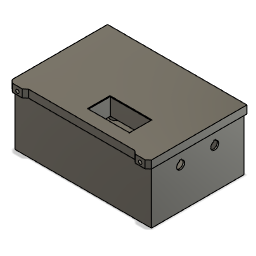
dcdc_ser_v5 (Autodesk Fusion 360 design; units mm, degrees)
Autodesk Fusion 360 part; units mm, degrees
sketch "Skizze1" plane through (0, 0, 0) normal (0, 1, 0) x (1, 0, 0)
  line L0 (0, 0) -> (100, 0) construction
  line L1 (100, 0) -> (100, -64) construction
  line L2 (100, -64) -> (0, -64) construction
  line L3 (0, -64) -> (0, 0) construction
  line L4 (0, 0) -> (100, -64) construction
  circle A0 centre (0, 0) radius 2
  circle A1 centre (0, 0) radius 5
  circle A2 centre (100, 0) radius 5
  circle A3 centre (100, 0) radius 2
  circle A4 centre (0, -64) radius 5
  circle A5 centre (0, -64) radius 2
  circle A6 centre (100, -64) radius 5
  circle A7 centre (100, -64) radius 2
  line L5 (-15, 14) -> (115, 14)
  line L6 (115, 14) -> (115, -78)
  line L7 (115, -78) -> (-15, -78)
  line L8 (-15, -78) -> (-15, 14)
  line L9 (-15, 14) -> (115, -78) construction
  line L10 (115, 14) -> (-15, -78) construction
  line L11 (116.5, -79.5) -> (-16.5, -79.5)
  line L12 (-16.5, -79.5) -> (-16.5, 15.5)
  line L13 (-16.5, 15.5) -> (116.5, 15.5)
  line L14 (116.5, 15.5) -> (116.5, -79.5)
  point P0 (50, -32)
  dimension "d1" = 100
  dimension "d2" = 64
  dimension "d3" = 4
  dimension "d4" = 10
  dimension "d7" = 100
  dimension "d8" = -64
  dimension "d9" = 130
  dimension "d10" = 92
  dimension "d11" = -1.5
  constraint horizontal L0
  constraint vertical L1
  constraint horizontal L2
  constraint vertical L3
  constraint coincident L0.start L3.end
  constraint horizontal L5
  constraint perpendicular L5 L6
  constraint parallel L5 L7
  constraint parallel L6 L8
  constraint coincident L9 P0
  constraint coincident L10 P0
  constraint midpoint L4 P0
  measures "d1" distance of L0.start L0.end
  measures "d2" distance of L0.start L2.end
  measures "d3" diameter of A0
  measures "d4" diameter of A1
  measures "d9" distance of L6.end L7.end
  measures "d10" distance of L5.end L6.end
extrude "Extrusion1" add sketch "Skizze1" against normal blind 1 contours A0 | A1 | A2 | A3 | A4 | A5 | A6 | A7 | L5 L6 L7 L8 | L11 L12 L13 L14 makes body 1
extrude "Extrusion2" add sketch "Skizze1" along normal blind 5 contours A1 | A2 | A4 | A6 bodies 1
extrude "Extrusion3" add sketch "Skizze1" along normal blind 60 contours L11 L12 L13 L14 bodies 1
sketch "Skizze2" plane through (116.5, 0, 0) normal (1, 0, 0) x (0, 0, -1)
  line L0 (-79.5, 60) -> (-79.5, -1)
  line L1 (-79.5, -1) -> (15.5, -1)
  line L2 (15.5, -1) -> (15.5, 60)
  line L3 (15.5, 60) -> (-79.5, 60)
  line L4 (-79.5, 60) -> (15.5, 60) construction
  line L5 (15.5, 60) -> (15.5, 40) construction
  line L6 (15.5, 40) -> (-79.5, 40) construction
  line L7 (-79.5, 40) -> (-79.5, 60) construction
  circle A0 centre (-32, 40) radius 17.5 construction
  line L8 (-49.5, 40) -> (-49.5, 44.1) construction
  line L9 (-14.5, 40) -> (-14.5, 44.1) construction
  line L10 (-48.5, 44.85) -> (-50.5, 44.85)
  line L11 (-50.5, 44.85) -> (-50.5, 43.35)
  line L12 (-49.5, 43.35) -> (-48.5, 43.35)
  line L13 (-48.5, 43.35) -> (-48.5, 44.85)
  line L14 (-48.5, 44.85) -> (-50.5, 43.35) construction
  line L15 (-50.5, 44.85) -> (-48.5, 43.35) construction
  line L16 (-13.5, 44.85) -> (-15.5, 44.85)
  line L17 (-15.5, 44.85) -> (-15.5, 43.35)
  line L18 (-14.8236, 43.35) -> (-13.5, 43.35)
  line L19 (-13.5, 43.35) -> (-13.5, 44.85)
  line L20 (-13.5, 44.85) -> (-15.5, 43.35) construction
  line L21 (-15.5, 44.85) -> (-13.5, 43.35) construction
  arc A1 (-50.5, 43.9762) -> (-49.5, 44.1) centre (-49.5, 40) ccw
  arc A2 (-15.5, 43.9762) -> (-14.9803, 44.0718) centre (-14.5, 40) ccw
  point P0 (-49.5, 44.1)
  point P1 (-14.5, 44.1)
  dimension "d18" = 20
  dimension "d19" = 35
  dimension "d20" = 8.2
  dimension "d21" = 8.2
  dimension "d22" = 2
  dimension "d23" = 1.5
  dimension "d24" = 2
  dimension "d25" = 1.5
  constraint horizontal L4
  constraint vertical L5
  constraint horizontal L6
  constraint vertical L7
  constraint coincident L2 L5.end
  constraint coincident L0.start L3.end
  constraint midpoint L6 A0.centre
  constraint coincident A0 L8.start
  constraint coincident L6 L8.start
  constraint coincident A0 L9.start
  constraint coincident L6 L9.start
  constraint coincident L8.start A1.centre
  constraint tangent A0 L8
  constraint perpendicular L6 L8
  constraint coincident L9.start A2.centre
  constraint coincident P1 A2
  constraint tangent A0 L9
  constraint perpendicular L6 L9
  constraint horizontal L10
  constraint perpendicular L10 L11
  constraint parallel L10 L12
  constraint parallel L11 L13
  constraint coincident L14 P0
  constraint coincident L15 P0
  constraint coincident P0 L8.end
  constraint horizontal L16
  constraint perpendicular L16 L17
  constraint parallel L16 L18
  constraint parallel L17 L19
  constraint coincident L20 P1
  constraint coincident L21 P1
  constraint coincident P1 L9.end
  constraint coincident L8 L12.start
  constraint coincident L11 A1.start
  constraint coincident A0 L18.start
  constraint coincident A0 A2.end
  constraint coincident L17 A2.start
  measures "d18" distance of L0.start L6.end
  measures "d19" diameter of A0
  measures "d20" diameter of A1
  measures "d21" diameter of A2
  measures "d22" distance of L11.end L12.end
  measures "d23" distance of L10.end L11.end
  measures "d24" distance of L17.end L18.end
  measures "d25" distance of L16.end L17.end
extrude "Extrusion4" cut sketch "Skizze2" against normal blind 6 contours L10 L11 L13 A1 | L16 L17 L19 A2 bodies 1
sketch "Skizze3" plane through (-16.5, 0, 0) normal (-1, 0, 0) x (0, 0, 1)
  line L0 (-15.5, 60) -> (-15.5, -1)
  line L1 (-15.5, -1) -> (79.5, -1)
  line L2 (79.5, -1) -> (79.5, 60)
  line L3 (79.5, 60) -> (-15.5, 60)
  line L4 (14.5, 40) -> (14.5, 44.1)
  circle A0 centre (14.5, 43.5) radius 1 construction
  line L5 (13.5103, 43.3571) -> (14.5, 44.5)
  line L6 (15.4897, 43.3571) -> (14.5, 44.5)
  arc A1 (13.5103, 43.3571) -> (14.5, 43.5) centre (14.5, 40) ccw
  arc A2 (13.5103, 23.3571) -> (14.5, 23.5) centre (14.5, 20) ccw
  line L7 (15.4897, 23.3571) -> (14.5, 24.5)
  line L8 (13.5103, 23.3571) -> (14.5, 24.5)
  line L9 (14.4549, 36.5003) -> (14.5, 23.5) construction
  line L10 (14.4774, 30.0001) -> (79.5, 30.0001) construction
  circle A3 centre (46.9887, 30.0001) radius 9
  line L11 (56.9887, 31.0001) -> (54.9887, 31.0001)
  line L12 (54.9887, 31.0001) -> (54.9887, 29.0001)
  line L13 (55.933, 29.0001) -> (56.9887, 29.0001)
  line L14 (56.9887, 29.0001) -> (56.9887, 31.0001)
  line L15 (56.9887, 31.0001) -> (54.9887, 29.0001) construction
  line L16 (54.9887, 31.0001) -> (56.9887, 29.0001) construction
  line L17 (38.0445, 29.0001) -> (36.9887, 29.0001)
  line L18 (36.9887, 29.0001) -> (36.9887, 31.0001)
  line L19 (36.9887, 31.0001) -> (38.9887, 31.0001)
  line L20 (38.9887, 31.0001) -> (38.9887, 29.0001)
  line L21 (38.9887, 29.0001) -> (36.9887, 31.0001) construction
  line L22 (36.9887, 29.0001) -> (38.9887, 31.0001) construction
  line L23 (38.0445, 29.0001) -> (38.9887, 29.9444)
  line L24 (55.933, 29.0001) -> (54.9887, 30.0001)
  point P0 (14.5, 40)
  point P1 (14.5, 44.1)
  point P2 (55.9887, 30.0001)
  point P3 (37.9887, 30.0001)
  dimension "d28" = 7
  dimension "d30" = 2
  dimension "d36" = 0
  dimension "d37" = -20
  dimension "d38" = 18
  dimension "d39" = 2
  dimension "d40" = 2
  dimension "d41" = 2
  dimension "d42" = 2
  constraint coincident P0 L4.start
  constraint coincident L4 A0.centre
  constraint coincident A0 L5.start
  constraint coincident A0 L5.end
  constraint coincident A0 L6.start
  constraint coincident L6.start A1
  constraint coincident A1 L9.start
  constraint midpoint L9 L10.start
  constraint coincident L2 L10.end
  constraint perpendicular L2 L10
  constraint midpoint L10 A3.centre
  constraint horizontal L11
  constraint perpendicular L11 L12
  constraint parallel L11 L13
  constraint parallel L12 L14
  constraint coincident L15 P2
  constraint coincident L16 P2
  constraint coincident A3 P2
  constraint coincident L10 P2
  constraint horizontal L17
  constraint perpendicular L17 L18
  constraint parallel L17 L19
  constraint parallel L18 L20
  constraint coincident L21 P3
  constraint coincident L22 P3
  constraint coincident L10 P3
  constraint coincident A3 P3
  constraint coincident A3 L17.start
  constraint coincident L20 L23.end
  constraint perpendicular L21 L23
  constraint coincident A3 L13.start
  constraint midpoint L12 L24.end
  measures "d28" diameter of A1
  measures "d30" diameter of A0
  measures "d38" diameter of A3
  measures "d39" distance of L12.end L13.end
  measures "d40" distance of L11.end L12.end
  measures "d41" distance of L18.end L19.end
  measures "d42" distance of L17.end L18.end
extrude "Extrusion6" cut sketch "Skizze3" against normal blind 3 contours L5 L6 A1 | A2 L7 L8 | A3 L11 L12 L19 L20 L23 L24 bodies 1
move_face "Flächen versetzen1" offset 7 1 faces at (-16.5, 26.6324, -6.6277) on bodies 1
move_face "Flächen versetzen2" offset -7 1 faces at (-15, 32.9593, -5.6051) on bodies 1
ref_plane "Arbeitsebene1" through (46.5, 60, 32) normal (0, 1, 0) x (0, 0, 1)
sketch "Skizze4" plane through (0, 60, 0) normal (0, 1, 0) x (1, 0, 0)
  line L0 (115, -78) -> (-22, -78)
  line L1 (-22, -78) -> (-22, 14)
  line L2 (-22, 14) -> (115, 14)
  line L3 (115, 14) -> (115, -78)
  line L4 (116.5, 15.5) -> (-23.5, 15.5)
  line L5 (-23.5, 15.5) -> (-23.5, -79.5)
  line L6 (-23.5, -79.5) -> (116.5, -79.5)
  line L7 (116.5, -79.5) -> (116.5, 15.5)
  line L8 (-23.7, -79.7) -> (116.7, -79.7)
  line L9 (116.7, -79.7) -> (116.7, 15.7)
  line L10 (116.7, 15.7) -> (-23.7, 15.7)
  line L11 (-23.7, 15.7) -> (-23.7, -79.7)
  line L12 (-25, -81) -> (118, -81)
  line L13 (118, -81) -> (118, 17)
  line L14 (118, 17) -> (-25, 17)
  line L15 (-25, 17) -> (-25, -81)
  line L16 (114.8, -77.8) -> (-21.8, -77.8)
  line L17 (-21.8, -77.8) -> (-21.8, 13.8)
  line L18 (-21.8, 13.8) -> (114.8, 13.8)
  line L19 (114.8, 13.8) -> (114.8, -77.8)
  line L20 (113.5, -76.5) -> (-20.5, -76.5)
  line L21 (-20.5, -76.5) -> (-20.5, 12.5)
  line L22 (-20.5, 12.5) -> (113.5, 12.5)
  line L23 (113.5, 12.5) -> (113.5, -76.5)
  dimension "d48" = 0.2
  dimension "d49" = 1.5
  dimension "d50" = 0.2
  dimension "d51" = 1.5
extrude "Extrusion7" add sketch "Skizze4" against normal blind 7 separate body contours L12 L13 L14 L15 | L16 L17 L18 L19 makes body 2 at (70.3333, 57.6667, -17) makes body 3 at (69.2667, 57.6667, 77.8)
extrude "Extrusion8" add sketch "Skizze4" along normal blind 1 contours L0 L1 L2 L3 | L4 L5 L6 L7 | L8 L9 L10 L11 | L12 L13 L14 L15 | L16 L17 L18 L19 | L20 L21 L22 L23 bodies 2 3
sketch "Skizze7" plane through (0, 61, 0) normal (0, 1, 0) x (-1, 0, 0)
  line L0 (25, -17) -> (25, 81)
  line L1 (25, 81) -> (-118, 81)
  line L2 (-118, 81) -> (-118, -17)
  line L3 (-118, -17) -> (25, -17)
  line L4 (-118, 81) -> (-61, 81) construction
  line L5 (-61, 81) -> (-61, 56.5) construction
  line L6 (-61, 56.5) -> (-118, 56.5) construction
  line L7 (-118, 56.5) -> (-118, 81) construction
  line L8 (-82.5, 68) -> (-39.5, 68)
  line L9 (-39.5, 68) -> (-39.5, 45)
  line L10 (-39.5, 45) -> (-82.5, 45)
  line L11 (-82.5, 45) -> (-82.5, 68)
  line L12 (-82.5, 68) -> (-39.5, 45) construction
  line L13 (-39.5, 68) -> (-82.5, 45) construction
  point P0 (-61, 56.5)
  dimension "d76" = 57
  dimension "d77" = 24.5
  dimension "d78" = 43
  dimension "d79" = 23
  constraint horizontal L4
  constraint vertical L5
  constraint horizontal L6
  constraint vertical L7
  constraint coincident L1.end L2.start
  constraint horizontal L8
  constraint perpendicular L8 L9
  constraint parallel L8 L10
  constraint parallel L9 L11
  constraint coincident L12 P0
  constraint coincident L13 P0
  constraint coincident P0 L5.end
  measures "d76" distance of L1.end L4.end
  measures "d77" distance of L1.end L6.end
  measures "d78" distance of L9.end L10.end
  measures "d79" distance of L8.end L9.end
extrude "Extrusion12" cut sketch "Skizze7" against normal blind 3 contours L8 L9 L10 L11 bodies 2
sketch "Skizze8" plane through (0, 60, 0) normal (0, -1, 0) x (1, 0, 0)
  line L0 (39.5, 45) -> (39.5, 68)
  line L1 (39.5, 68) -> (82.5, 68)
  line L2 (82.5, 68) -> (82.5, 45)
  line L3 (82.5, 45) -> (39.5, 45)
  line L4 (113.5, -12.5) -> (113.5, 76.5)
  line L5 (113.5, 76.5) -> (-20.5, 76.5)
  line L6 (-20.5, 76.5) -> (-20.5, -12.5)
  line L7 (-20.5, -12.5) -> (113.5, -12.5)
  line L8 (39.5, 68) -> (82.5, 45) construction
  line L9 (85, 70.95) -> (37, 70.95)
  line L10 (37, 70.95) -> (37, 42.05)
  line L11 (37, 42.05) -> (85, 42.05)
  line L12 (85, 42.05) -> (85, 70.95)
  line L13 (85, 70.95) -> (37, 42.05) construction
  line L14 (37, 70.95) -> (85, 42.05) construction
  line L15 (35, 40.05) -> (87, 40.05)
  line L16 (87, 40.05) -> (87, 72.95)
  line L17 (87, 72.95) -> (35, 72.95)
  line L18 (35, 72.95) -> (35, 40.05)
  line L19 (-20.5, -12.5) -> (34.7443, 39.8079)
  line L20 (-19.1249, -13.9523) -> (36.4539, 38.6724)
  line L21 (-19.3935, 78.166) -> (35, 42.039)
  line L22 (37.9947, 40.05) -> (114.6065, -10.834)
  line L23 (-20.5, 76.5) -> (34.7443, 39.8079)
  line L24 (36.4539, 38.6724) -> (113.5, -12.5)
  point P0 (61, 56.5)
  dimension "d82" = 48
  dimension "d83" = 28.9
  dimension "d84" = 2
  constraint coincident L0.end L1.start
  constraint coincident L2.end L3.start
  constraint horizontal L9
  constraint perpendicular L9 L10
  constraint parallel L9 L11
  constraint parallel L10 L12
  constraint coincident L13 P0
  constraint coincident L14 P0
  constraint midpoint L8 P0
  constraint coincident L5.end L6.start
  constraint coincident L4.start L7.end
  constraint coincident L6.end L7.start
  constraint coincident L18 L21.end
  constraint coincident L15 L22.start
  constraint collinear L21 L22
  constraint coincident L20.end L23
  constraint collinear L23 L24
  measures "d82" distance of L10.end L11.end
  measures "d83" distance of L9.end L10.end
extrude "Extrusion13" add sketch "Skizze8" along normal blind 20 contours L15 L16 L17 L18 bodies 2
extrude "Extrusion14" add sketch "Skizze8" along normal blind 4 contours L4 L5 L7 L15 L18 L19 L20 L21 L22 L23 L24 bodies 2
chamfer "Fase2" distance 3 angle 45 4 edges at (62.4973, 60, 40.05) (87, 60, 56.5) (35, 60, 57.4945) (61, 60, 72.95) on bodies 2
sketch "Skizze9" plane through (0, 0, 81) normal (0, 0, 1) x (1, 0, 0)
  line L0 (-25, 61) -> (-25, 53)
  line L1 (-25, 53) -> (118, 53)
  line L2 (118, 53) -> (118, 61)
  line L3 (118, 61) -> (-25, 61)
  line L4 (118, 53) -> (113, 53) construction
  line L5 (113, 53) -> (113, 59.5773) construction
  line L6 (113, 59.5773) -> (118, 59.5773) construction
  line L7 (118, 59.5773) -> (118, 53) construction
  line L8 (113, 59.5773) -> (106, 59.5773) construction
  line L9 (106, 59.5773) -> (106, 53) construction
  line L10 (106, 53) -> (113, 53) construction
  line L11 (113, 53) -> (113, 59.5773) construction
  line L12 (106, 59.5773) -> (106.3441, 59.5773) construction
  line L13 (106, 59.5773) -> (113, 53) construction
  circle A0 centre (109.5, 56.2887) radius 1.75
  line L14 (114.5, 61.3386) -> (104.5, 61.3386)
  line L15 (104.5, 61.3386) -> (104.5, 51.2388)
  line L16 (104.5, 51.2388) -> (114.5, 51.2388)
  line L17 (114.5, 51.2388) -> (114.5, 61.3386)
  line L18 (114.5, 61.3386) -> (104.5, 51.2388) construction
  line L19 (104.5, 61.3386) -> (114.5, 51.2388) construction
  line L20 (109.5, 56.2887) -> (-26, 56.2887) construction
  line L21 (-25, 56.2887) -> (-16.5, 56.2887) construction
  circle A1 centre (-16.5, 56.2887) radius 1.75
  line L22 (-11.5, 61) -> (-21.5, 61)
  line L23 (-21.5, 61) -> (-21.5, 51.5773)
  line L24 (-21.5, 51.5773) -> (-11.5, 51.5773)
  line L25 (-11.5, 51.5773) -> (-11.5, 61)
  line L26 (-11.5, 61) -> (-21.5, 51.5773) construction
  line L27 (-21.5, 61) -> (-11.5, 51.5773) construction
  point P0 (109.5, 56.2887)
  point P1 (-16.5, 56.2887)
  dimension "d92" = 5
  dimension "d93" = 3.5
  dimension "d94" = 10
  dimension "d95" = 8.5
  dimension "d96" = 3.5
  dimension "d97" = 10
  constraint horizontal L4
  constraint vertical L5
  constraint horizontal L6
  constraint vertical L7
  constraint coincident L1.end L2.start
  constraint horizontal L8
  constraint vertical L9
  constraint horizontal L10
  constraint vertical L11
  constraint coincident L1 L9.end
  constraint coincident L8 L12.end
  constraint midpoint L13 P0
  constraint horizontal L14
  constraint perpendicular L14 L15
  constraint parallel L14 L16
  constraint parallel L15 L17
  constraint coincident L18 P0
  constraint coincident L19 P0
  constraint coincident P0 A0.centre
  constraint perpendicular L0 L20
  constraint coincident L20 L21.start
  constraint coincident L0 L21.start
  constraint perpendicular L0 L21
  constraint coincident P1 L21.end
  constraint horizontal L22
  constraint perpendicular L22 L23
  constraint parallel L22 L24
  constraint parallel L23 L25
  constraint coincident L26 P1
  constraint coincident L27 P1
  constraint coincident L3 L22.start
  measures "d92" distance of L1.end L4.end
  measures "d93" diameter of A0
  measures "d94" distance of L15.end L16.end
  measures "d95" distance of L21.start P1
  measures "d96" diameter of A1
  measures "d97" distance of L23.end L24.end
extrude "Extrusion15" add sketch "Skizze9" along normal blind 3 contours L1 L3 L22 L23 L25 | L1 L3 L15 L17 bodies 2
extrude "Extrusion16" cut sketch "Skizze9" against normal blind 2 contours A0 | A1 bodies 2
chamfer "Fase3" distance 3.5 distance2 3 4 edges at (-11.5, 57, 81) (114.5, 57, 81) (-21.5, 57, 81) (104.5, 57, 81) measured on face at (27.1667, 58.3333, 81) measured on face at (115.6667, 58.3333, 81) measured on face at (-22.6667, 58.3333, 81) measured on face at (27.1667, 58.3333, 81) on bodies 2
sketch "Skizze5" plane through (0, 61, 0) normal (0, 1, 0) x (-1, 0, 0)
  line L0 (25, -17) -> (25, 81)
  line L1 (25, 81) -> (-118, 81)
  line L2 (-118, 81) -> (-118, -17)
  line L3 (-118, -17) -> (25, -17)
  line L4 (-118, 81) -> (-46.5, 81) construction
  line L5 (-46.5, 81) -> (-46.5, 32) construction
  line L6 (-46.5, 32) -> (-118, 32) construction
  line L7 (-118, 32) -> (-118, 81) construction
  line L8 (-46.5, 32) -> (-118, 81) construction
  line L9 (-82.25, 56.5) -> (-81, 56.5)
  line L10 (-81, 56.5) -> (-61, 56.5)
  line L11 (-39.5, 68) -> (-82.5, 68)
  line L12 (-82.5, 68) -> (-82.5, 45)
  line L13 (-82.5, 45) -> (-39.5, 45)
  line L14 (-39.5, 45) -> (-39.5, 68)
  line L15 (-39.5, 68) -> (-82.5, 45) construction
  line L16 (-82.5, 68) -> (-39.5, 45) construction
  point P0 (-82.25, 56.5)
  point P1 (-61, 56.5)
  dimension "d56" = 71.5
  dimension "d57" = 49
  dimension "d73" = 20
  dimension "d74" = 43
  dimension "d75" = 23
  constraint horizontal L4
  constraint vertical L5
  constraint horizontal L6
  constraint vertical L7
  constraint coincident L1.end L2.start
  constraint midpoint L8 P0
  constraint coincident P0 L9.start
  constraint horizontal L9
  constraint parallel L9 L10
  constraint horizontal L11
  constraint perpendicular L11 L12
  constraint parallel L11 L13
  constraint parallel L12 L14
  constraint coincident L15 P1
  constraint coincident L16 P1
  constraint coincident P1 L10.end
  measures "d56" distance of L1.end L4.end
  measures "d57" distance of L1.end L6.end
  measures "d73" distance of L9.end P1
  measures "d74" distance of L12.end L13.end
  measures "d75" distance of L11.end L12.end
extrude "Extrusion9" [suppressed]
sketch "Skizze6" plane through (0, 60, 0) normal (0, -1, 0) x (1, 0, 0)
  line L0 (60.75, 68) -> (103.75, 68)
  line L1 (103.75, 68) -> (103.75, 45)
  line L2 (103.75, 45) -> (60.75, 45)
  line L3 (60.75, 45) -> (60.75, 68)
  line L4 (113.5, -12.5) -> (113.5, 76.5)
  line L5 (113.5, 76.5) -> (-20.5, 76.5)
  line L6 (-20.5, 76.5) -> (-20.5, -12.5)
  line L7 (-20.5, -12.5) -> (113.5, -12.5)
  line L8 (60.75, 45) -> (103.75, 68) construction
  line L9 (106.25, 42.05) -> (58.25, 42.05)
  line L10 (58.25, 42.05) -> (58.25, 70.95)
  line L11 (58.25, 70.95) -> (106.25, 70.95)
  line L12 (106.25, 70.95) -> (106.25, 42.05)
  line L13 (106.25, 42.05) -> (58.25, 70.95) construction
  line L14 (58.25, 42.05) -> (106.25, 70.95) construction
  line L15 (108.25, 40.05) -> (56.25, 40.05)
  line L16 (56.25, 40.05) -> (56.25, 72.95)
  line L17 (56.25, 72.95) -> (108.25, 72.95)
  line L18 (108.25, 72.95) -> (108.25, 40.05)
  line L19 (108.25, 72.95) -> (113.5, 76.5)
  line L20 (108.25, 70.5357) -> (114.6203, 74.8432)
  line L21 (-20.5, 76.5) -> (45.4812, 32.6767)
  line L22 (47.2781, 31.4832) -> (113.5, -12.5)
  line L23 (-19.3701, -14.1502) -> (45.4982, 30.2644)
  line L24 (47.2781, 31.4832) -> (59.7901, 40.05)
  line L25 (-20.5, -12.5) -> (43.7012, 31.458)
  line L26 (45.4812, 32.6767) -> (56.25, 40.05)
  line L27 (-21.6065, 74.834) -> (43.7012, 31.458)
  line L28 (45.4982, 30.2644) -> (112.3935, -14.166)
  point P0 (82.25, 56.5)
  dimension "d62" = 48
  dimension "d63" = 28.9
  dimension "d64" = -2
  constraint coincident L2.end L3.start
  constraint coincident L0.end L1.start
  constraint horizontal L9
  constraint perpendicular L9 L10
  constraint parallel L9 L11
  constraint parallel L10 L12
  constraint coincident L13 P0
  constraint coincident L14 P0
  constraint midpoint L8 P0
  constraint coincident L5.end L6.start
  constraint coincident L4.start L7.end
  constraint coincident L6.end L7.start
  constraint coincident L4.end L5.start
  constraint coincident L18 L20.start
  constraint coincident L15 L24.end
  constraint coincident L21.end L25
  constraint coincident L22.start L23
  constraint collinear L21 L22
  constraint coincident L23.end L27
  constraint collinear L23 L24
  constraint collinear L25 L26
  constraint collinear L27 L28
  measures "d62" distance of L10.end L11.end
  measures "d63" distance of L9.end L10.end
extrude "Extrusion10" [suppressed]
extrude "Extrusion11" [suppressed]
chamfer "Fase1" [suppressed]
extrude "Extrusion5" [suppressed]
named bodies: "Unterteil", "Oberteil"
